Autodesk Inventor part; units mm, degrees
(part 2 of 2)
  line L757 (-609.0008, 1017.8823) -> (-649.9584, 1046.5611)
  line L758 (-649.9584, 1046.5611) -> (-621.2796, 1087.5187)
  line L759 (-621.2796, 1087.5187) -> (-580.322, 1058.8399)
  line L760 (-580.322, 1058.8399) -> (-609.0008, 1017.8823)
  line L761 (-662.2457, 1055.1648) -> (-703.2033, 1083.8436)
  line L762 (-703.2033, 1083.8436) -> (-674.5244, 1124.8012)
  line L763 (-674.5244, 1124.8012) -> (-633.5668, 1096.1224)
  line L764 (-633.5668, 1096.1224) -> (-662.2457, 1055.1648)
  line L765 (-715.4905, 1092.4472) -> (-756.4481, 1121.126)
  line L766 (-756.4481, 1121.126) -> (-727.7693, 1162.0836)
  line L767 (-727.7693, 1162.0836) -> (-686.8117, 1133.4048)
  line L768 (-686.8117, 1133.4048) -> (-715.4905, 1092.4472)
  line L769 (-768.7354, 1129.7297) -> (-809.693, 1158.4085)
  line L770 (-809.693, 1158.4085) -> (-781.0142, 1199.3661)
  line L771 (-781.0142, 1199.3661) -> (-740.0566, 1170.6873)
  line L772 (-740.0566, 1170.6873) -> (-768.7354, 1129.7297)
  line L773 (-821.9803, 1167.0122) -> (-862.9379, 1195.691)
  line L774 (-862.9379, 1195.691) -> (-834.2591, 1236.6486)
  line L775 (-834.2591, 1236.6486) -> (-793.3015, 1207.9698)
  line L776 (-793.3015, 1207.9698) -> (-821.9803, 1167.0122)
  line L777 (-875.2252, 1204.2946) -> (-916.1828, 1232.9734)
  line L778 (-916.1828, 1232.9734) -> (-887.504, 1273.9311)
  line L779 (-887.504, 1273.9311) -> (-846.5464, 1245.2522)
  line L780 (-846.5464, 1245.2522) -> (-875.2252, 1204.2946)
  line L781 (-167.0793, 629.0952) -> (-208.0369, 657.774)
  line L782 (-208.0369, 657.774) -> (-179.3581, 698.7316)
  line L783 (-179.3581, 698.7316) -> (-138.4005, 670.0528)
  line L784 (-138.4005, 670.0528) -> (-167.0793, 629.0952)
  line L785 (-220.3242, 666.3777) -> (-261.2818, 695.0565)
  line L786 (-261.2818, 695.0565) -> (-232.603, 736.0141)
  line L787 (-232.603, 736.0141) -> (-191.6454, 707.3353)
  line L788 (-191.6454, 707.3353) -> (-220.3242, 666.3777)
  line L789 (-273.5691, 703.6601) -> (-314.5267, 732.3389)
  line L790 (-314.5267, 732.3389) -> (-285.8478, 773.2965)
  line L791 (-285.8478, 773.2965) -> (-244.8902, 744.6177)
  line L792 (-244.8902, 744.6177) -> (-273.5691, 703.6601)
  line L793 (-326.8139, 740.9426) -> (-367.7715, 769.6214)
  line L794 (-367.7715, 769.6214) -> (-339.0927, 810.579)
  line L795 (-339.0927, 810.579) -> (-298.1351, 781.9002)
  line L796 (-298.1351, 781.9002) -> (-326.8139, 740.9426)
  line L797 (-380.0588, 778.2251) -> (-421.0164, 806.9039)
  line L798 (-421.0164, 806.9039) -> (-392.3376, 847.8615)
  line L799 (-392.3376, 847.8615) -> (-351.38, 819.1827)
  line L800 (-351.38, 819.1827) -> (-380.0588, 778.2251)
  line L801 (-433.3037, 815.5075) -> (-474.2613, 844.1863)
  line L802 (-474.2613, 844.1863) -> (-445.5825, 885.144)
  line L803 (-445.5825, 885.144) -> (-404.6249, 856.4651)
  line L804 (-404.6249, 856.4651) -> (-433.3037, 815.5075)
  line L805 (-486.5486, 852.79) -> (-527.5062, 881.4688)
  line L806 (-527.5062, 881.4688) -> (-498.8274, 922.4264)
  line L807 (-498.8274, 922.4264) -> (-457.8698, 893.7476)
  line L808 (-457.8698, 893.7476) -> (-486.5486, 852.79)
  line L809 (-539.7935, 890.0725) -> (-580.7511, 918.7513)
  line L810 (-580.7511, 918.7513) -> (-552.0723, 959.7089)
  line L811 (-552.0723, 959.7089) -> (-511.1147, 931.0301)
  line L812 (-511.1147, 931.0301) -> (-539.7935, 890.0725)
  line L813 (-593.0384, 927.3549) -> (-633.996, 956.0338)
  line L814 (-633.996, 956.0338) -> (-605.3171, 996.9914)
  line L815 (-605.3171, 996.9914) -> (-564.3595, 968.3125)
  line L816 (-564.3595, 968.3125) -> (-593.0384, 927.3549)
  line L817 (-646.2832, 964.6374) -> (-687.2408, 993.3162)
  line L818 (-687.2408, 993.3162) -> (-658.562, 1034.2738)
  line L819 (-658.562, 1034.2738) -> (-617.6044, 1005.595)
  line L820 (-617.6044, 1005.595) -> (-646.2832, 964.6374)
  line L821 (-699.5281, 1001.9199) -> (-740.4857, 1030.5987)
  line L822 (-740.4857, 1030.5987) -> (-711.8069, 1071.5563)
  line L823 (-711.8069, 1071.5563) -> (-670.8493, 1042.8775)
  line L824 (-670.8493, 1042.8775) -> (-699.5281, 1001.9199)
  line L825 (-752.773, 1039.2023) -> (-793.7306, 1067.8812)
  line L826 (-793.7306, 1067.8812) -> (-765.0518, 1108.8388)
  line L827 (-765.0518, 1108.8388) -> (-724.0942, 1080.1599)
  line L828 (-724.0942, 1080.1599) -> (-752.773, 1039.2023)
  line L829 (-806.0179, 1076.4848) -> (-846.9755, 1105.1636)
  line L830 (-846.9755, 1105.1636) -> (-818.2967, 1146.1212)
  line L831 (-818.2967, 1146.1212) -> (-777.3391, 1117.4424)
  line L832 (-777.3391, 1117.4424) -> (-806.0179, 1076.4848)
  line L833 (-859.2628, 1113.7673) -> (-900.2204, 1142.4461)
  line L834 (-900.2204, 1142.4461) -> (-871.5416, 1183.4037)
  line L835 (-871.5416, 1183.4037) -> (-830.584, 1154.7249)
  line L836 (-830.584, 1154.7249) -> (-859.2628, 1113.7673)
  line L837 (-912.5077, 1151.0497) -> (-953.4653, 1179.7286)
  line L838 (-953.4653, 1179.7286) -> (-924.7864, 1220.6862)
  line L839 (-924.7864, 1220.6862) -> (-883.8288, 1192.0073)
  line L840 (-883.8288, 1192.0073) -> (-912.5077, 1151.0497)
  line L841 (-204.3618, 575.8503) -> (-245.3194, 604.5291)
  line L842 (-245.3194, 604.5291) -> (-216.6405, 645.4867)
  line L843 (-216.6405, 645.4867) -> (-175.6829, 616.8079)
  line L844 (-175.6829, 616.8079) -> (-204.3618, 575.8503)
  line L845 (-257.6066, 613.1328) -> (-298.5642, 641.8116)
  line L846 (-298.5642, 641.8116) -> (-269.8854, 682.7692)
  line L847 (-269.8854, 682.7692) -> (-228.9278, 654.0904)
  line L848 (-228.9278, 654.0904) -> (-257.6066, 613.1328)
  line L849 (-310.8515, 650.4152) -> (-351.8091, 679.0941)
  line L850 (-351.8091, 679.0941) -> (-323.1303, 720.0517)
  line L851 (-323.1303, 720.0517) -> (-282.1727, 691.3728)
  line L852 (-282.1727, 691.3728) -> (-310.8515, 650.4152)
  line L853 (-364.0964, 687.6977) -> (-405.054, 716.3765)
  line L854 (-405.054, 716.3765) -> (-376.3752, 757.3341)
  line L855 (-376.3752, 757.3341) -> (-335.4176, 728.6553)
  line L856 (-335.4176, 728.6553) -> (-364.0964, 687.6977)
  line L857 (-417.3413, 724.9802) -> (-458.2989, 753.659)
  line L858 (-458.2989, 753.659) -> (-429.6201, 794.6166)
  line L859 (-429.6201, 794.6166) -> (-388.6625, 765.9378)
  line L860 (-388.6625, 765.9378) -> (-417.3413, 724.9802)
  line L861 (-470.5862, 762.2626) -> (-511.5438, 790.9415)
  line L862 (-511.5438, 790.9415) -> (-482.865, 831.8991)
  line L863 (-482.865, 831.8991) -> (-441.9074, 803.2202)
  line L864 (-441.9074, 803.2202) -> (-470.5862, 762.2626)
  line L865 (-523.8311, 799.5451) -> (-564.7887, 828.2239)
  line L866 (-564.7887, 828.2239) -> (-536.1098, 869.1815)
  line L867 (-536.1098, 869.1815) -> (-495.1522, 840.5027)
  line L868 (-495.1522, 840.5027) -> (-523.8311, 799.5451)
  line L869 (-577.0759, 836.8276) -> (-618.0335, 865.5064)
  line L870 (-618.0335, 865.5064) -> (-589.3547, 906.464)
  line L871 (-589.3547, 906.464) -> (-548.3971, 877.7852)
  line L872 (-548.3971, 877.7852) -> (-577.0759, 836.8276)
  line L873 (-630.3208, 874.1101) -> (-671.2784, 902.7889)
  line L874 (-671.2784, 902.7889) -> (-642.5996, 943.7465)
  line L875 (-642.5996, 943.7465) -> (-601.642, 915.0677)
  line L876 (-601.642, 915.0677) -> (-630.3208, 874.1101)
  line L877 (-683.5657, 911.3925) -> (-724.5233, 940.0713)
  line L878 (-724.5233, 940.0713) -> (-695.8445, 981.0289)
  line L879 (-695.8445, 981.0289) -> (-654.8869, 952.3501)
  line L880 (-654.8869, 952.3501) -> (-683.5657, 911.3925)
  line L881 (-736.8106, 948.675) -> (-777.7682, 977.3538)
  line L882 (-777.7682, 977.3538) -> (-749.0894, 1018.3114)
  line L883 (-749.0894, 1018.3114) -> (-708.1318, 989.6326)
  line L884 (-708.1318, 989.6326) -> (-736.8106, 948.675)
  line L885 (-790.0555, 985.9575) -> (-831.0131, 1014.6363)
  line L886 (-831.0131, 1014.6363) -> (-802.3343, 1055.5939)
  line L887 (-802.3343, 1055.5939) -> (-761.3767, 1026.9151)
  line L888 (-761.3767, 1026.9151) -> (-790.0555, 985.9575)
  line L889 (-843.3004, 1023.2399) -> (-884.258, 1051.9187)
  line L890 (-884.258, 1051.9187) -> (-855.5791, 1092.8763)
  line L891 (-855.5791, 1092.8763) -> (-814.6215, 1064.1975)
  line L892 (-814.6215, 1064.1975) -> (-843.3004, 1023.2399)
  line L893 (-896.5452, 1060.5224) -> (-937.5028, 1089.2012)
  line L894 (-937.5028, 1089.2012) -> (-908.824, 1130.1588)
  line L895 (-908.824, 1130.1588) -> (-867.8664, 1101.48)
  line L896 (-867.8664, 1101.48) -> (-896.5452, 1060.5224)
  line L897 (-949.7901, 1097.8049) -> (-990.7477, 1126.4837)
  line L898 (-990.7477, 1126.4837) -> (-962.0689, 1167.4413)
  line L899 (-962.0689, 1167.4413) -> (-921.1113, 1138.7625)
  line L900 (-921.1113, 1138.7625) -> (-949.7901, 1097.8049)
  line L901 (-360, 1580) -> (-360, 980) projected
  line L902 (-360, 980) -> (-660, 980) projected
  line L903 (-660, 980) -> (-660, 1580) projected
  line L904 (-660, 1580) -> (-360, 1580) projected
  line L905 (-320, 1580) -> (-20, 1580) projected
  line L906 (-20, 1580) -> (-20, 980) projected
  line L907 (-20, 980) -> (-320, 980) projected
  line L908 (-320, 980) -> (-320, 1580) projected
  line L909 (0, 900) -> (0, 1610) projected
  line L910 (0, 1610) -> (-715, 1610) projected
  line L911 (-715, 1610) -> (-715, 900) projected
  line L912 (0, 900) -> (-715, 900) projected
  point P0 (0, 0)
  point P1 (-20, 1446.039)
  point P2 (-20, 1464.3506)
  point P3 (-25.5588, 1485)
  point P4 (-43.8704, 1485)
  point P5 (-49.4904, 1485)
  point P6 (-75.6421, 1485)
  point P7 (-104.9091, 1485)
  point P8 (-123.2207, 1485)
  point P9 (-162.8144, 1485)
  point P10 (-202.5711, 1485)
  point P11 (-197.0901, 1580)
  point P12 (-302.2901, 1485)
  point P13 (-320, 1436.3618)
  point P14 (-320, 1404.4665)
  point P15 (-320, 1357.0115)
  point P16 (-320, 1338.6999)
  point P17 (-320, 1317.2941)
  point P18 (-320, 1291.1424)
  point P19 (-320, 1277.6612)
  point P20 (-320, 1259.3495)
  point P21 (-320, 1203.9701)
  point P22 (-320, 1177.8184)
  point P23 (-320, 1118.9605)
  point P24 (-320, 1100.6488)
  point P25 (-320, 1090.646)
  point P26 (-320, 1064.4943)
  point P27 (-320, 1039.6101)
  point P28 (-320, 1021.2985)
  point P29 (-320, 977.322)
  point P30 (-320, 941.9481)
  point P31 (-305.2942, 885)
  point P32 (-286.9826, 885)
  point P33 (-238.6696, 885)
  point P34 (-141.1125, 980)
  point P35 (-146.5935, 885)
  point P36 (-128.2819, 885)
  point P37 (-125.3456, 885)
  point P38 (-99.1939, 885)
  point P39 (-67.2432, 885)
  point P40 (-48.9315, 885)
  point P41 (-20, 890.5866)
  point P42 (-20, 908.8982)
  point P43 (-20, 926.3185)
  point P44 (-20, 952.4702)
  point P45 (-20, 969.9369)
  point P46 (-20, 988.2485)
  point P47 (-20, 1039.6426)
  point P48 (-20, 1067.5989)
  point P49 (-20, 1128.6376)
  point P50 (-20, 1146.9492)
  point P51 (-20, 1152.9666)
  point P52 (-20, 1179.1183)
  point P53 (-20, 1207.988)
  point P54 (-20, 1226.2996)
  point P55 (-20, 1266.2907)
  point P56 (-20, 1305.6499)
  point P57 (-20, 1366.6887)
  point P58 (-20, 1405.7664)
  point P59 (-360, 1446.0585)
  point P60 (-361.2718, 1485)
  point P61 (-389.4625, 1485)
  point P62 (-415.6142, 1485)
  point P63 (-422.3105, 1485)
  point P64 (-440.6221, 1485)
  point P65 (-435.1411, 1580)
  point P66 (-528.9382, 1485)
  point P67 (-581.0112, 1485)
  point P68 (-532.8031, 1580)
  point P69 (-616.1106, 1485)
  point P70 (-642.2623, 1485)
  point P71 (-660, 1436.3814)
  point P72 (-660, 1418.0697)
  point P73 (-660, 1398.344)
  point P74 (-660, 1372.1923)
  point P75 (-660, 1357.031)
  point P76 (-660, 1338.7194)
  point P77 (-660, 1285.02)
  point P78 (-660, 1258.8683)
  point P79 (-660, 1198.3303)
  point P80 (-660, 1180.0187)
  point P81 (-660, 1171.6959)
  point P82 (-660, 1145.5442)
  point P83 (-660, 1118.98)
  point P84 (-660, 1100.6684)
  point P85 (-660, 1058.3719)
  point P86 (-660, 1021.318)
  point P87 (-660, 960.2793)
  point P88 (-660, 918.8961)
  point P89 (-622.6956, 885)
  point P90 (-604.384, 885)
  point P91 (-578.6418, 885)
  point P92 (-552.4901, 885)
  point P93 (-476.8255, 980)
  point P94 (-525.0336, 885)
  point P95 (-465.3177, 885)
  point P96 (-439.166, 885)
  point P97 (-384.6446, 885)
  point P98 (-366.3329, 885)
  point P99 (-360, 890.6061)
  point P100 (-360, 920.1961)
  point P101 (-360, 969.9564)
  point P102 (-360, 988.2681)
  point P103 (-360, 1007.3684)
  point P104 (-360, 1033.5201)
  point P105 (-360, 1049.3068)
  point P106 (-360, 1067.6184)
  point P107 (-360, 1120.6925)
  point P108 (-360, 1146.9688)
  point P109 (-360, 1208.0075)
  point P110 (-360, 1226.3191)
  point P111 (-360, 1234.0165)
  point P112 (-360, 1260.1682)
  point P113 (-360, 1287.3578)
  point P114 (-360, 1305.6695)
  point P115 (-360, 1347.3405)
  point P116 (-360, 1385.0198)
  point P117 (-127.7548, 980)
  point P118 (-241.0788, 980)
  point P119 (-62.0067, 920)
  point P120 (-61.7622, 980)
  point P121 (-24.4243, 920)
  point P122 (-78.0513, 1580)
  point P123 (-117.7397, 1580)
  point P124 (-191.3753, 1580)
  point P125 (-20, 1492.9387)
  point P126 (-20, 1519.0904)
  point P127 (-38.3894, 1580)
  point P128 (-320, 1497.4006)
  point P129 (-360.1373, 920)
  point P130 (-581.051, 980)
  point P131 (-617.2146, 980)
  point P132 (-375.8271, 920)
  point P133 (-401.9788, 920)
  point P134 (-379.1636, 980)
  point P135 (-578.9234, 1520)
  point P136 (-593.8418, 1580)
  point P137 (-660, 1485.5163)
  point P138 (-418.0234, 1580)
  point P139 (-360, 1486.8163)
  point P140 (-397.8032, 1520)
  point P141 (-537.8643, 980)
  point P142 (-20, 1478.3133)
  point P143 (-20, 1492.9387)
  point P144 (-660, 1485.5163)
  point P145 (-660, 1450.3441)
  point P146 (-20, 1539.3521)
  point P147 (-20, 1557.6637)
  point P148 (-136.0514, 1580)
  point P149 (-165.2236, 1580)
  point P150 (-215.4017, 1580)
  point P151 (-276.4404, 1580)
  point P152 (-304.6994, 1580)
  point P153 (-320, 1543.9422)
  point P154 (-320, 1511.3633)
  point P155 (-320, 1450.3246)
  point P156 (-320, 1432.0129)
  point P157 (-320, 1430.6182)
  point P158 (-320, 1404.4665)
  point P159 (-320, 1370.9742)
  point P160 (-320, 1352.6626)
  point P161 (-320, 1317.2941)
  point P162 (-320, 1273.3122)
  point P163 (-320, 1212.2735)
  point P164 (-320, 1177.8184)
  point P165 (-320, 1132.9232)
  point P166 (-320, 1114.6115)
  point P167 (-320, 1090.646)
  point P168 (-320, 1064.4943)
  point P169 (-320, 1053.5728)
  point P170 (-320, 1035.2612)
  point P171 (-318.1248, 980)
  point P172 (-299.8132, 980)
  point P173 (-214.9271, 980)
  point P174 (-159.4241, 980)
  point P175 (-101.6031, 980)
  point P176 (-80.0738, 980)
  point P177 (-20, 983.8996)
  point P178 (-20, 1002.2112)
  point P179 (-20, 1039.6426)
  point P180 (-20, 1081.5616)
  point P181 (-20, 1142.6003)
  point P182 (-20, 1179.1183)
  point P183 (-20, 1221.9507)
  point P184 (-20, 1240.2623)
  point P185 (-20, 1266.2907)
  point P186 (-20, 1292.4424)
  point P187 (-20, 1301.301)
  point P188 (-20, 1319.6126)
  point P189 (-20, 1379.6147)
  point P190 (-20, 1405.7664)
  point P191 (-20, 1460.0017)
  point P192 (-20, 1519.0904)
  point P193 (-360, 1539.3716)
  point P194 (-360, 1557.6832)
  point P195 (-360, 1573.9886)
  point P196 (-374.1024, 1580)
  point P197 (-391.8717, 1580)
  point P198 (-453.4528, 1580)
  point P199 (-505.1957, 1580)
  dimension "d68" = 50
  dimension "d69" = 50
  dimension "d70" = 35
  dimension "d73" = 65
  dimension "d76" = 65
  constraints: 1800 end point, 2 collinear, 2 parallel, 1 perpendicular, 1800 other
  measures "d68" distance of L0.start L0.end
  measures "d69" distance of L0.end L1.end
  measures "d70" angle to the sketch x axis of L0
  measures "d73" distance of L0.start L5.start
  measures "d76" distance of L0.start L61.start
extrude "Extrusion5" add sketch "Sketch3" along normal blind 2 and the other way blind 20 contours L4 L688 L687 L686 L685 L752 L751 L750 L815 L814 L820 L819 L818 L903 L764 L763 L701 L704 L703 L702 L708 L707 L645 L648 L647 L646 L589 L592 L591 L529 L532 L531 L530 L536 L535 L473 L476 L475 L474 L417 L420 L419 L904 L357 L360 L354 L353 L356 L289 L292 L286 L285 L288 L287 L225 L228 L901 L222 L221 L283 L282 L281 L284 L339 L338 L337 L399 L398 L397 L400 L394 L393 L455 L454 L453 L456 L511 L510 L509 L566 L565 L627 L626 L625 L628 L622 L621 L683 L682 | L624 L623 L908 L561 L564 L563 L562 L568 L567 L505 L508 L507 L506 L449 L452 L451 L396 L395 L333 L336 L335 L334 L340 L339 L277 L280 L279 L224 L223 L905 L158 L157 L160 L154 L153 L156 L155 L93 L96 L90 L89 L92 L91 L26 L25 L906 L87 L86 L85 L88 L82 L81 L143 L142 L141 L144 L198 L197 L259 L258 L257 L260 L254 L253 L315 L314 L313 L316 L371 L370 L369 L426 L425 L487 L486 L907 L492 L491 L490 L489 L551 L550 L556 L555 L554 L553 L619 L618
chamfer "Chamfer1" distance 30 angle 45 2 edges at (-390, 70, -900) (-815, 70, -865)
chamfer "Chamfer2" distance 30 angle 45 2 edges at (-787.5, 40, -490) (-810, 40, -55)
sketch "Sketch5" plane through (-715, 0, -1610) normal (-1, 0, 0) x (0, 0, 1)
  line L0 (0, 0) -> (0, 40) projected
  line L1 (0, 40) -> (-50, 8)
  line L2 (-50, 8) -> (-50, 0)
  line L3 (-50, 0) -> (0, 0)
  point P0 (1610, 0)
  dimension "d89" = 50
  dimension "d90" = 8
  constraints: 6 end point, 1 parallel, 1 perpendicular
  measures "d89" distance between parallel lines of L0 L2
  measures "d90" distance of L1.end L2.end
extrude "Extrusion6" add sketch "Sketch5" against normal up to surface (715 mm away)
sketch "Sketch6" plane through (-850, 0, 0) normal (0, 0, 1) x (1, 0, 0)
  line L0 (0, 20) -> (10, 20)
  line L1 (10, 20) -> (10, 50)
  line L2 (10, 50) -> (0, 50)
  line L3 (0, 50) -> (0, 20)
  line L4 (0, 0) -> (0, 70) projected
  line L5 (0, 0) -> (85, 0) projected
  circle A0 centre (5, 50) radius 3
  circle A1 centre (5, 20) radius 3
  point P0 (850, 0)
  point P1 (8, 50)
  point P2 (2, 50)
  point P3 (2, 20)
  point P4 (8, 20)
  dimension "d93" = 10
  dimension "d94" = 20
  dimension "d95" = 30
  dimension "d96" = 6
  dimension "d97" = 6
  constraints: 8 end point, 2 centre point, 2 midpoint, 2 parallel, 1 collinear, 1 horizontal, 1 perpendicular
  measures "d93" distance between parallel lines of L3 L1
  measures "d94" distance between parallel lines of L5 L0
  measures "d95" distance between parallel lines of L0 L2
  measures "d96" diameter of A0
  measures "d97" diameter of A1
extrude "Extrusion7" cut sketch "Sketch6" against normal through all contours A1 L0 L3 L2 A0 L1
mirror "Mirror1" about plane through (0, 0, 0) normal (1, 0, 0) of "Extrusion1", "Extrusion3", "Extrusion4", "Extrusion5", "Chamfer1", "Chamfer2", "Extrusion6", "Extrusion7"
equation "\"d65\" = d60"
body "Solid1"
